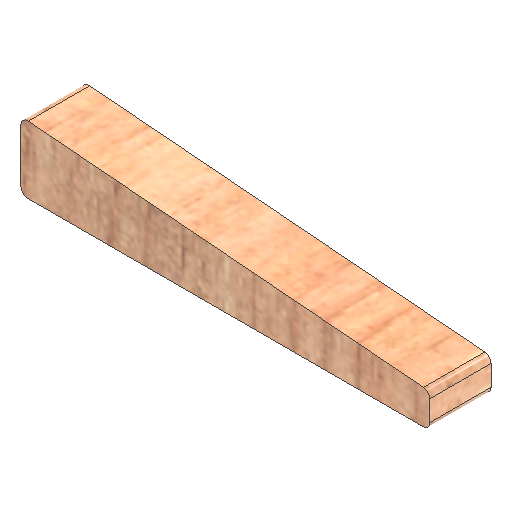
# Autodesk Inventor part: Wedge
Saved by Autodesk Inventor 2021 (Build 250183000, 183)
## iProperties
Created: 2020-05-09
Part Number: Wedge
Material: Wood (Birch)
Document SubType Name: Modeling
Designer: Dan Wikman
Density: 0.55 g/cm^3
Appearance: Birch - Natural Polished
Mass: 17.6669 g
Surface Area: 83.7066 cm^2
Volume: 32.1217 cm^3
Autodesk Inventor part; units mm, degrees
ref_plane "YZ Plane" through (0, 0, 0) normal (1, 0, 0) x (0, 1, 0)
ref_plane "XZ Plane" through (0, 0, 0) normal (0, 1, 0) x (-1, 0, 0)
ref_plane "XY Plane" through (0, 0, 0) normal (0, 0, 1) x (1, 0, 0)
sketch "CONTOURS" plane through (0, 0, 0) normal (0, 0, 1) x (1, 0, 0)
  line L0 (25, 917.9541) -> (25, 902.2281)
  arc A0 (25, 902.2281) -> (27, 900.2277) centre (27, 902.2277) ccw
  line L1 (27, 900.2277) -> (143, 900.2277)
  arc A1 (143, 900.2277) -> (145, 902.2277) centre (143, 902.2277) ccw
  line L2 (145, 902.2277) -> (145, 908.2874)
  arc A2 (145, 908.2874) -> (143.1661, 910.2805) centre (143, 908.2874) ccw
  line L3 (143.1661, 910.2805) -> (27.1661, 919.9472)
  arc A3 (27.1661, 919.9472) -> (25, 917.9541) centre (27, 917.9541) ccw
  constraints: 8 end point, 8 point on circle, 4 centre point
extrude "Extrusion1" add sketch "CONTOURS" along normal blind 18
body "Solid1"
